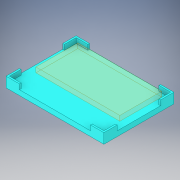
# Autodesk Inventor part: LCD-128X64BK_AG
Saved by Autodesk Inventor 2017.3 (Build 213256000, 256)
## iProperties
Part Number: LCD-128X64BK_AG
Material: Generisch
Document SubType Name: Modeling
Designer: Nils
Density: 1 g/cm^3
Appearance: LCD-128X64BK_AG, LCD-128X64BK_AG
Author: Nils
Autodesk Inventor part; units mm, degrees
ref_plane "YZ Plane" through (0, 0, 0) normal (1, 0, 0) x (0, 1, 0)
ref_plane "XZ Plane" through (0, 0, 0) normal (0, 1, 0) x (-1, 0, 0)
ref_plane "XY Plane" through (0, 0, 0) normal (0, 0, 1) x (1, 0, 0)
sketch "LCD-128X64BK_AG, LCD-128X64BK_AG_48" plane through (0, 0, 0) normal (0, 0, 1) x (1, 0, 0)
  line L0 (-29.1635, 20.0635) -> (29.1635, 20.0635)
  line L1 (29.1635, 20.0635) -> (29.1635, -21.7)
  line L2 (29.1635, -21.7) -> (-29.1635, -21.7)
  line L3 (-29.1635, -21.7) -> (-29.1635, 20.0635)
  constraints: 8 end point
extrude "Extrusion1" add sketch "LCD-128X64BK_AG, LCD-128X64BK_AG_48" along normal blind 3
sketch "Skizze2" plane through (0, 0, 3) normal (0, 0, 1) x (1, 0, 0)
  line L0 (29.1635, 20.0635) -> (-29.1635, 20.0635) construction
  line L1 (-29.1635, 20.0635) -> (-29.1635, -21.7) construction
  line L2 (-29.1635, -21.7) -> (29.1635, -21.7) construction
  line L3 (29.1635, -21.7) -> (29.1635, 20.0635) construction
  line L4 (-29.1635, 20.0635) -> (-29.1635, -21.7) projected
  line L5 (-29.1635, 20.0635) -> (-29.1635, 12.0635)
  line L6 (-29.1635, 12.0635) -> (-28.1635, 12.0635)
  line L7 (-28.1635, 12.0635) -> (-28.1635, 19.0635)
  line L8 (-28.1635, 19.0635) -> (-21.1635, 19.0635)
  line L9 (-21.1635, 19.0635) -> (-21.1635, 20.0635)
  line L10 (29.1635, 20.0635) -> (-29.1635, 20.0635) projected
  line L11 (-29.1635, 20.0635) -> (-21.1635, 20.0635)
  line L12 (-29.1635, -21.7) -> (-21.1635, -21.7)
  line L13 (-29.1635, -21.7) -> (29.1635, -21.7) projected
  line L14 (-21.1635, -21.7) -> (-21.1635, -20.7)
  line L15 (-21.1635, -20.7) -> (-28.1635, -20.7)
  line L16 (-28.1635, -20.7) -> (-28.1635, -13.7)
  line L17 (-28.1635, -13.7) -> (-29.1635, -13.7)
  line L18 (-29.1635, -21.7) -> (-29.1635, -13.7)
  line L19 (29.1635, -21.7) -> (29.1635, 20.0635) projected
  line L20 (29.1635, -21.7) -> (21.1635, -21.7)
  line L21 (21.1635, -21.7) -> (21.1635, -20.7)
  line L22 (21.1635, -20.7) -> (28.1635, -20.7)
  line L23 (28.1635, -20.7) -> (28.1635, -13.7)
  line L24 (28.1635, -13.7) -> (29.1635, -13.7)
  line L25 (29.1635, -21.7) -> (29.1635, -13.7)
  line L26 (21.1635, 20.0635) -> (29.1635, 20.0635)
  line L27 (29.1635, 20.0635) -> (29.1635, 12.0635)
  line L28 (28.1635, 12.0635) -> (28.1635, 19.0635)
  line L29 (28.1635, 19.0635) -> (21.1635, 19.0635)
  line L30 (21.1635, 19.0635) -> (21.1635, 20.0635)
  line L31 (28.1635, 12.0635) -> (29.1635, 12.0635)
  point P0 (0, 0)
  dimension "d2" = 8
  dimension "d3" = 1
  dimension "d4" = 7
  dimension "d5" = 7
  dimension "d6" = 8
  dimension "d7" = 1
  dimension "d8" = 7
  dimension "d9" = 7
  dimension "d10" = 8
  dimension "d11" = 1
  dimension "d12" = 7
  dimension "d13" = 7
  dimension "d14" = 8
  dimension "d15" = 8
  dimension "d16" = 7
  dimension "d17" = 7
  constraints: 48 end point, 15 point on line, 7 perpendicular, 4 collinear, 2 vertical, 1 horizontal, 1 parallel
  measures "d2" distance of L0.end L5.end
  measures "d3" distance of L5.end L6.end
  measures "d4" distance of L6.end L7.end
  measures "d5" distance of L7.end L8.end
  measures "d6" distance of L1.end L12.end
  measures "d7" distance of L12.end L14.end
  measures "d8" distance of L14.end L15.end
  measures "d9" distance of L15.end L16.end
  measures "d10" distance of L2.end L20.end
  measures "d11" distance of L20.end L21.end
  measures "d12" distance of L21.end L22.end
  measures "d13" distance of L22.end L23.end
  measures "d14" distance of L26.start L0.start
  measures "d15" distance between parallel lines of L26 L31
  measures "d16" distance of L28.end L29.end
  measures "d17" distance of L28.start L28.end
extrude "Extrusion2" add sketch "Skizze2" along normal blind 3 contours L10 L9 L8 L7 L6 L4 | L17 L16 L15 L14 L12 L4 | L10 L19 L31 L28 L29 L30 | L21 L22 L23 L24 L19 L13
sketch "Skizze3" plane through (0, 0, 3) normal (0, 0, 1) x (1, 0, 0)
  line L0 (-25, 16.9635) -> (25, 16.9635)
  line L1 (25, 16.9635) -> (25, -8.0365)
  line L2 (25, -8.0365) -> (-25, -8.0365)
  line L3 (-25, -8.0365) -> (-25, 16.9635)
  line L4 (-40.8289, 0) -> (40.8289, 0) construction
  line L5 (0, -30.0527) -> (0, 28.4162) construction
  line L6 (-21.1635, -20.7) -> (-21.1635, -21.7) construction
  line L7 (-21.1635, -21.7) -> (21.1635, -21.7) construction
  line L8 (21.1635, -21.7) -> (21.1635, -20.7) construction
  line L9 (21.1635, -20.7) -> (28.1635, -20.7) construction
  line L10 (28.1635, -20.7) -> (28.1635, -13.7) construction
  line L11 (28.1635, -13.7) -> (29.1635, -13.7) construction
  line L12 (29.1635, -13.7) -> (29.1635, 12.0635) construction
  line L13 (29.1635, 12.0635) -> (28.1635, 12.0635) construction
  line L14 (28.1635, 12.0635) -> (28.1635, 19.0635) construction
  line L15 (28.1635, 19.0635) -> (21.1635, 19.0635) construction
  line L16 (21.1635, 19.0635) -> (21.1635, 20.0635) construction
  line L17 (21.1635, 20.0635) -> (-21.1635, 20.0635) construction
  line L18 (-21.1635, 20.0635) -> (-21.1635, 19.0635) construction
  line L19 (-21.1635, 19.0635) -> (-28.1635, 19.0635) construction
  line L20 (-28.1635, 19.0635) -> (-28.1635, 12.0635) construction
  line L21 (-28.1635, 12.0635) -> (-29.1635, 12.0635) construction
  line L22 (-29.1635, 12.0635) -> (-29.1635, -13.7) construction
  line L23 (-29.1635, -13.7) -> (-28.1635, -13.7) construction
  line L24 (-28.1635, -13.7) -> (-28.1635, -20.7) construction
  line L25 (-28.1635, -20.7) -> (-21.1635, -20.7) construction
  point P0 (0, 0)
  point P1 (0, 16.9635)
  dimension "d20" = 3.1
  dimension "d21" = 25
  dimension "d22" = 50
  constraints: 8 end point, 2 parallel, 1 horizontal, 1 midpoint, 1 perpendicular, 1 point on line
  measures "d20" distance between parallel lines of L17 L0
  measures "d21" distance of L2.end L0.start
  measures "d22" distance of L0.start L0.end
extrude "Extrusion3" add sketch "Skizze3" along normal blind 3 separate body
